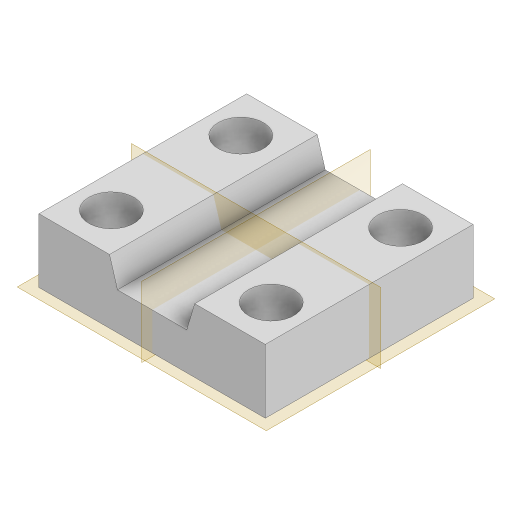
# Autodesk Inventor part: Крепление мотора2
Saved by Autodesk Inventor 2023.2 (Build 272271030, 271C)
## iProperties
Created: 2024-12-17
Part Number: Крепление мотора2
Material: Типовые
Document SubType Name: Modeling
Designer: I9232
Density: 1 g/cm^3
Appearance: По умолчанию
Author: I9232
Autodesk Inventor part; units mm, degrees
sketch "Эскиз1" plane through (0, 0, 0) normal (0, 1, 0) x (-1, 0, 0)
  line L0 (21.25, 19.5) -> (-21.25, 19.5)
  line L1 (-21.25, 19.5) -> (-21.25, -19.5)
  line L2 (-21.25, -19.5) -> (21.25, -19.5)
  line L3 (21.25, -19.5) -> (21.25, 19.5)
  line L4 (21.25, 19.5) -> (-21.25, -19.5) construction
  line L5 (-21.25, 19.5) -> (21.25, -19.5) construction
  circle A0 centre (-15, -12.15) radius 4.25
  line L6 (0, -19.5) -> (0, 19.5) construction
  line L7 (-21.25, 0) -> (21.25, 0) construction
  circle A1 centre (15, -12.15) radius 4.25
  circle A2 centre (-15, 12.15) radius 4.25
  circle A3 centre (15, 12.15) radius 4.25
  point P0 (0, 0)
  dimension "d0" = 39
  dimension "d1" = 42.5
  dimension "d2" = 8.5
  dimension "d3" = 6.25
  dimension "d4" = 7.35
  constraints: 16 end point, 6 midpoint, 4 centre point, 3 symmetric about line, 2 parallel, 1 horizontal, 1 perpendicular, 3 other
  measures "d0" distance of L0.end L1.end
  measures "d1" distance of L1.end L2.end
  measures "d2" diameter of A0
  measures "d3" distance from line of L1 A0.centre
  measures "d4" distance from line of L2 A0.centre
extrude "Выдавливание1" add sketch "Эскиз1" along normal blind 12
sketch "Эскиз2" plane through (-21.25, 0, 19.5) normal (0, 0, 1) x (1, 0, 0)
  line L0 (14.75, 7) -> (27.75, 7)
  line L1 (0, 12) -> (42.5, 12) projected
  line L2 (13.25, 12) -> (29.25, 12)
  line L3 (21.25, 14.4) -> (21.25, -2.4) construction
  line L4 (13.25, 12) -> (14.75, 7)
  line L5 (29.25, 12) -> (27.75, 7)
  point P0 (21.25, 0)
  point P1 (21.25, 12)
  point P2 (21.25, 7)
  point P3 (13.25, 12)
  dimension "d7" = 13
  dimension "d8" = 5
  dimension "d9" = 16
  constraints: 8 end point, 2 horizontal, 2 midpoint, 2 point on line, 1 collinear
  measures "d7" distance of L0.start L0.end
  measures "d8" distance between parallel lines of L0 L1
  measures "d9" distance of L2.start L2.end
extrude "Выдавливание2" cut sketch "Эскиз2" against normal up to surface (39 mm away)
